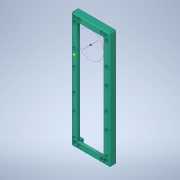
# Autodesk Inventor part: 10_Lid_1x1_v2
Saved by Autodesk Inventor 2022.3 (Build 263350000, 350)
## iProperties
Created: 2019-07-01
Part Number: 10_Lid_1x1_v2
Material: Generic
Document SubType Name: Modeling
Designer: diederichbenedict
Density: 1 g/cm^3
Appearance: IPHT_Türkis
Author: diederichbenedict
Autodesk Inventor part; units mm, degrees
ref_plane "Work Plane1" through (0, 41.8, -12.9) normal (0, 0, 1) x (1, 0, 0)
sketch "Sketch1" plane through (0, 41.8, -12.9) normal (0, 0, 1) x (1, 0, 0)
  line L0 (3.85, 0.3752) -> (3.85, 4) construction
  line L1 (3.85, 4) -> (-2, 4) construction
  arc A0 (-2, 4) -> (-4, 2) centre (-2, 2) ccw construction
  line L2 (-4, 2) -> (-4, -3.85) construction
  line L3 (-4, -3.85) -> (-0.3752, -3.85) construction
  line L4 (-2, 4) -> (43.8, 4)
  line L5 (45.8, 2) -> (45.8, -43.8)
  line L6 (-4, -43.8) -> (-4, 2)
  line L7 (40.3, -37.8) -> (40.3, -4)
  line L8 (37.8, -1.5) -> (4, -1.5)
  line L9 (1.5, -4) -> (1.5, -37.8)
  line L10 (4, -1.5) -> (1.5, -4)
  line L11 (40.3, -4) -> (37.8, -1.5)
  arc A1 (45.8, 2) -> (43.8, 4) centre (43.8, 2) ccw
  arc A2 (-2, 4) -> (-4, 2) centre (-2, 2) ccw
  circle A3 centre (1, -1) radius 1.4
  circle A4 centre (40.8, -1) radius 1.4
  circle A5 centre (40.8, -40.8) radius 1.4 construction
  circle A6 centre (1, -40.8) radius 1.4 construction
  circle A7 centre (20.9, -20.9) radius 19.4 construction
  line L12 (3.85, -3.85) -> (3.85, -37.95)
  line L13 (37.95, -37.95) -> (37.95, -3.85)
  line L14 (37.95, -3.85) -> (3.85, -3.85)
  arc A8 (2.2654, -1.2094) -> (1.2094, -2.2654) centre (0.9, -0.9) ccw projected
  line L15 (2.2654, -1.2094) -> (3.85, 0.3752) projected
  line L16 (-0.3752, -3.85) -> (1.2094, -2.2654) projected
  line L17 (45.8, -47.8) -> (45.8, -93.6)
  line L18 (-4, -93.6) -> (-4, -47.8)
  line L19 (40.3, -87.6) -> (40.3, -53.8)
  line L20 (1.5, -53.8) -> (1.5, -87.6)
  line L21 (40.3, -53.8) -> (37.95, -51.45)
  circle A9 centre (1, -50.8) radius 1.4 construction
  circle A10 centre (40.8, -50.7733) radius 1.4 construction
  circle A11 centre (40.8, -90.6) radius 1.4 construction
  circle A12 centre (1, -90.6) radius 1.4 construction
  circle A13 centre (20.9, -70.7) radius 19.4 construction
  line L22 (3.85, -53.65) -> (3.85, -87.75)
  line L23 (37.95, -87.75) -> (37.95, -53.65)
  line L24 (45.8, -97.6) -> (45.8, -143.4)
  line L25 (43.8, -145.4) -> (-2, -145.4)
  line L26 (-4, -143.4) -> (-4, -97.6)
  line L27 (40.3, -137.4) -> (40.3, -103.6)
  line L28 (1.5, -103.6) -> (1.5, -137.4)
  line L29 (4, -139.9) -> (37.8, -139.9)
  line L30 (37.8, -139.9) -> (40.3, -137.4)
  line L31 (4, -139.9) -> (1.5, -137.4)
  line L32 (40.3, -103.6) -> (37.95, -101.25)
  arc A14 (43.8, -145.4) -> (45.8, -143.4) centre (43.8, -143.4) ccw
  arc A15 (-4, -143.4) -> (-2, -145.4) centre (-2, -143.4) ccw
  circle A16 centre (1, -100.6) radius 1.4 construction
  circle A17 centre (40.8, -100.5154) radius 1.4 construction
  circle A18 centre (40.8, -140.4) radius 1.4
  circle A19 centre (1, -140.4) radius 1.4
  circle A20 centre (20.9, -120.5) radius 19.4 construction
  line L33 (3.85, -103.45) -> (3.85, -137.55)
  line L34 (3.85, -137.55) -> (37.95, -137.55)
  line L35 (37.95, -137.55) -> (37.95, -103.45)
  line L36 (37.95, -37.95) -> (37.95, -40.15)
  line L37 (3.85, -61.4449) -> (3.85, -51.45)
  line L38 (37.95, -37.95) -> (37.95, -40.15)
  line L39 (3.85, -53.65) -> (3.85, -51.45)
  line L40 (3.85, -40.15) -> (3.85, -37.95)
  line L41 (37.95, -40.15) -> (40.3, -37.8)
  line L42 (3.85, -51.45) -> (3.85, -40.15)
  line L43 (3.85, -51.45) -> (3.85, -40.15)
  line L44 (-4, -43.8) -> (-4, -47.8)
  line L45 (45.8, -43.8) -> (45.8, -47.8)
  line L46 (3.85, -40.15) -> (3.85, -37.95)
  line L47 (3.85, -51.45) -> (3.85, -45.8)
  line L48 (37.95, -51.45) -> (37.95, -53.65)
  line L49 (37.95, -40.15) -> (37.95, -51.45)
  line L50 (3.85, -40.15) -> (1.5, -37.8)
  line L51 (3.85, -51.45) -> (1.5, -53.8)
  line L52 (37.95, -40.15) -> (37.95, -51.45)
  line L53 (37.95, -51.45) -> (37.95, -53.65)
  line L54 (37.95, -87.75) -> (37.95, -89.95)
  line L55 (3.85, -87.75) -> (3.85, -89.95)
  line L56 (3.85, -89.95) -> (3.85, -101.25)
  line L57 (3.85, -101.25) -> (1.5, -103.6)
  line L58 (3.85, -101.25) -> (3.85, -103.45)
  line L59 (3.85, -89.95) -> (1.5, -87.6)
  line L60 (37.95, -89.95) -> (37.95, -101.25)
  line L61 (37.95, -89.95) -> (40.3, -87.6)
  line L62 (37.95, -101.25) -> (37.95, -103.45)
  line L63 (-4, -93.6) -> (-4, -97.6)
  line L64 (45.8, -93.6) -> (45.8, -97.6)
  point P0 (45.8, -45.8)
  point P1 (45.8, 4)
  point P2 (-4, -45.8)
  point P3 (40.3, -40.3)
  point P4 (40.3, -1.5)
  point P5 (1.5, -1.5)
  point P6 (1.5, -40.3)
  point P7 (40.8, -1)
  point P8 (45.8, -95.6)
  point P9 (45.8, -45.8)
  point P10 (-4, -95.6)
  point P11 (40.3, -90.1)
  point P12 (40.3, -51.3)
  point P13 (1.5, -51.3)
  point P14 (1.5, -90.1)
  point P15 (40.8, -50.8)
  point P16 (45.8, -145.4)
  point P17 (45.8, -95.6)
  point P18 (-4, -145.4)
  point P19 (40.3, -139.9)
  point P20 (40.3, -101.1)
  point P21 (1.5, -101.1)
  point P22 (1.5, -139.9)
  point P23 (40.8, -100.6)
  point P24 (-0.0387, -1.9387)
  point P25 (1.9387, 0.0387)
  dimension "d55" = 2.8
  dimension "d34" = 49.8
  dimension "d35" = 49.8
  dimension "d36" = 5.5
  dimension "d38" = 2.5
  dimension "d40" = 2.5
  dimension "d41" = 2.5
  dimension "d42" = 2.5
  dimension "d43" = 2.5
  dimension "d44" = 2.5
  dimension "d45" = 2
  dimension "d46" = 5
  dimension "d48" = 5
  dimension "d51" = 5
  dimension "d52" = 0.5
  dimension "d53" = 5
  dimension "d54" = 5
  dimension "d56" = 2.8
  dimension "d57" = 2.8
  dimension "d58" = 2.8
  dimension "d90" = 7.85
  dimension "d112" = 49.8
  dimension "d113" = 49.8
  dimension "d114" = 5.5
  dimension "d116" = 2.5
  dimension "d118" = 2.5
  dimension "d120" = 2.5
  dimension "d121" = 2.5
  dimension "d124" = 5
  dimension "d126" = 5
  dimension "d129" = 0.5
  dimension "d130" = 2.8
  dimension "d131" = 2.8
  dimension "d132" = 2.8
  dimension "d133" = 2.8
  dimension "d134" = 7.85
  dimension "d135" = 49.8
  dimension "d136" = 49.8
  dimension "d137" = 5.5
  dimension "d138" = 2.5
  dimension "d139" = 2.5
  dimension "d140" = 2.5
  dimension "d141" = 2.5
  dimension "d143" = 2.5
  dimension "d144" = 2.5
  dimension "d147" = 5
  dimension "d148" = 5
  dimension "d149" = 5
  dimension "d150" = 5
  dimension "d152" = 0.5
  dimension "d153" = 2.8
  dimension "d154" = 2.8
  dimension "d155" = 2.8
  dimension "d156" = 2.8
  dimension "d157" = 7.85
  constraints: 118 end point, 30 parallel, 30 point on line, 17 centre point, 13 tangent, 9 coincident, 8 point on circle, 4 collinear, 3 perpendicular, 2 vertical, 1 equal radius, 1 horizontal, 1 midpoint, 11 other
  measures "d34" distance of point (45.8, -45.8) point (-4, -45.8)
  measures "d35" distance of point (45.8, 4) point (45.8, -45.8)
  measures "d36" distance between parallel lines of L5 L7
  measures "d38" distance of L7.start point (40.3, -40.3)
  measures "d40" distance of L9.end point (1.5, -40.3)
  measures "d41" distance of L8.end point (1.5, -1.5)
  measures "d42" distance of L9.start point (1.5, -1.5)
  measures "d43" distance of L7.end point (40.3, -1.5)
  measures "d44" distance of L8.start point (40.3, -1.5)
  measures "d45" radius of A1
  measures "d46" distance from line of point (1, -40.8) L6
  measures "d48" distance from line of L5 point (40.8, -40.8)
  measures "d51" distance from line of L4 point (40.8, -1)
  measures "d52" distance from line of point (1, -1) L9
  measures "d53" distance from line of L2 point (1, -1)
  measures "d54" distance from line of L1 point (1, -1)
  measures "d56" diameter of A4
  measures "d57" diameter of A5
  measures "d58" diameter of A6
  measures "d90" distance between parallel lines of L6 L12
  measures "d112" distance of point (45.8, -95.6) point (-4, -95.6)
  measures "d113" distance of point (45.8, -45.8) point (45.8, -95.6)
  measures "d114" distance between parallel lines of L17 L19
  measures "d116" distance of L19.start point (40.3, -90.1)
  measures "d118" distance of L20.end point (1.5, -90.1)
  measures "d120" distance of L20.start point (1.5, -51.3)
  measures "d121" distance of L19.end point (40.3, -51.3)
  measures "d124" distance from line of point (1, -90.6) L18
  measures "d126" distance from line of L17 point (40.8, -90.6)
  measures "d129" distance from line of point (1, -50.8) L20
  measures "d130" diameter of A9
  measures "d131" diameter of A10
  measures "d132" diameter of A11
  measures "d133" diameter of A12
  measures "d134" distance between parallel lines of L18 L22
  measures "d135" distance of point (45.8, -145.4) point (-4, -145.4)
  measures "d136" distance of point (45.8, -95.6) point (45.8, -145.4)
  measures "d137" distance between parallel lines of L24 L27
  measures "d138" distance of L29.end point (40.3, -139.9)
  measures "d139" distance of L27.start point (40.3, -139.9)
  measures "d140" distance of L29.start point (1.5, -139.9)
  measures "d141" distance of L31.end point (1.5, -139.9)
  measures "d143" distance of L28.start point (1.5, -101.1)
  measures "d144" distance of L27.end point (40.3, -101.1)
  measures "d147" distance from line of point (1, -140.4) L26
  measures "d148" distance from line of L25 point (1, -140.4)
  measures "d149" distance from line of L24 point (40.8, -140.4)
  measures "d150" distance from line of L25 point (40.8, -140.4)
  measures "d152" distance from line of point (1, -100.6) L28
  measures "d153" diameter of A16
  measures "d154" diameter of A17
  measures "d155" diameter of A18
  measures "d156" diameter of A19
  measures "d157" distance between parallel lines of L26 L33
extrude "Extrusion1" add sketch "Sketch1" along normal blind 7.7 contours L4 A1 L5 L45 L17 L64 L24 A14 L25 A15 L26 L63 L18 L44 L6 A2 | L41 L36 L13 L14 L12 L40 L50 L9 L10 L8 L11 L7 | L21 L19 L61 L54 L23 L48 | L32 L27 L30 L29 L31 L28 L57 L58 L33 L34 L35 L62 | L37 L22 L55 L59 L20 L51
fillet "Fillet1" radius 2 5 edges at (45.8, -28.9, -5.2) (45.2142, 45.2142, -5.2) (20.9, 45.8, -5.2) (-3.4142, 45.2142, -5.2) (-4, -28.9, -5.2)
sketch "Sketch2" plane through (-2, -4, -12.9) normal (0, -1, 0) x (1, 0, 0)
  line L0 (43.8, -4.8712) -> (42.35, -4)
  line L1 (2, -4.8712) -> (0.55, -4)
  line L2 (-2, 0) -> (-2, 5.7) construction
  line L3 (45.8, 7.7) -> (0, 7.7) construction
  line L4 (47.8, 0) -> (47.8, 5.7) construction
  circle A0 centre (2.9, -62.2) radius 1.45 projected
  line L5 (9.4548, -67.1) -> (36.3452, -67.1) projected
  point P0 (2, 12.9)
  point P1 (2.9, 2.8)
  point P2 (42.9, 2.8)
  dimension "d59" = 4.9
  dimension "d60" = 4.9
  dimension "d61" = 4.9
  dimension "d62" = 4.9
  constraints: 4 end point, 6 other
  measures "d59" distance from line of point (2.9, 2.8) L2
  measures "d60" distance from line of point (2.9, 2.8) L3
  measures "d61" distance from line of point (42.9, 2.8) L4
  measures "d62" distance from line of point (42.9, 2.8) L3
hole "Hole1" [suppressed]
sketch "Sketch3" plane through (0, 41.8, -5.2) normal (0, 0, 1) x (1, 0, 0)
  circle A0 centre (20.9, -20.9) radius 16.9 construction
  point P0 (0, -41.8)
  constraints: 1 centre point
sketch "Sketch4" plane through (0, 41.8, -5.2) normal (0, 0, 1) x (1, 0, 0)
  line L0 (37.95, -37.95) -> (37.95, -3.85) projected
  line L1 (37.95, -3.85) -> (3.85, -3.85) projected
  line L2 (3.85, -3.85) -> (3.85, -37.95) projected
  line L3 (3.85, -37.95) -> (37.95, -37.95) projected
  circle A0 centre (40.9, -0.9) radius 2.75 projected
  circle A1 centre (0.9, -40.9) radius 2.75 projected
  circle A2 centre (0.9, -0.9) radius 2.75 projected
  circle A3 centre (40.9, -40.9) radius 2.75 projected
  line L4 (34.3452, 2) -> (7.4548, 2) projected
  line L5 (43.8, -34.3452) -> (43.8, -7.4548) projected
  line L6 (7.4548, -43.8) -> (34.3452, -43.8) projected
  line L7 (-2, -7.4548) -> (-2, -34.3452) projected
  arc A4 (34.3452, 2) -> (36.4548, 2) centre (35.4, -0.1) ccw projected
  line L8 (43.8, 2) -> (36.4548, 2) projected
  line L9 (43.8, -5.3452) -> (43.8, 2) projected
  arc A5 (43.8, -5.3452) -> (43.8, -7.4548) centre (41.7, -6.4) ccw projected
  arc A6 (43.8, -34.3452) -> (43.8, -36.4548) centre (41.7, -35.4) ccw projected
  line L10 (43.8, -43.8) -> (43.8, -36.4548) projected
  line L11 (36.4548, -43.8) -> (43.8, -43.8) projected
  arc A7 (36.4548, -43.8) -> (34.3452, -43.8) centre (35.4, -41.7) ccw projected
  arc A8 (7.4548, -43.8) -> (5.3452, -43.8) centre (6.4, -41.7) ccw projected
  line L12 (-2, -43.8) -> (5.3452, -43.8) projected
  line L13 (-2, -36.4548) -> (-2, -43.8) projected
  arc A9 (-2, -36.4548) -> (-2, -34.3452) centre (0.1, -35.4) ccw projected
  arc A10 (-2, -7.4548) -> (-2, -5.3452) centre (0.1, -6.4) ccw projected
  line L14 (-2, 2) -> (-2, -5.3452) projected
  line L15 (5.3452, 2) -> (-2, 2) projected
  arc A11 (5.3452, 2) -> (7.4548, 2) centre (6.4, -0.1) ccw projected
  line L16 (37.9698, -87.8712) -> (37.9698, -53.7712)
  line L17 (37.9698, -53.7712) -> (3.8698, -53.7712)
  line L18 (3.8698, -53.7712) -> (3.8698, -87.8712)
  line L19 (3.8698, -87.8712) -> (37.9698, -87.8712)
  circle A12 centre (40.9, -50.8212) radius 2.75
  circle A13 centre (0.9, -90.8212) radius 2.75
  circle A14 centre (0.9, -50.8212) radius 2.75
  circle A15 centre (40.9198, -90.8212) radius 2.75
  line L20 (34.3651, -47.7932) -> (7.4746, -47.7932)
  line L21 (43.8198, -84.1385) -> (43.8198, -57.248)
  line L22 (7.4746, -93.5932) -> (34.3651, -93.5932)
  line L23 (-1.9802, -57.248) -> (-1.9802, -84.1385)
  arc A16 (34.3651, -47.7932) -> (36.4746, -47.7932) centre (35.4198, -49.8932) ccw
  line L24 (43.8198, -47.7932) -> (36.4746, -47.7932)
  line L25 (43.8198, -55.1385) -> (43.8198, -47.7932)
  arc A17 (43.8198, -55.1385) -> (43.8198, -57.248) centre (41.7198, -56.1932) ccw
  arc A18 (43.8198, -84.1385) -> (43.8198, -86.248) centre (41.7198, -85.1932) ccw
  line L26 (43.8198, -93.5932) -> (43.8198, -86.248)
  line L27 (36.4746, -93.5932) -> (43.8198, -93.5932)
  arc A19 (36.4746, -93.5932) -> (34.3651, -93.5932) centre (35.4198, -91.4932) ccw
  arc A20 (7.4746, -93.5932) -> (5.3651, -93.5932) centre (6.4198, -91.4932) ccw
  line L28 (-1.9802, -93.5932) -> (5.3651, -93.5932)
  line L29 (-1.9802, -86.248) -> (-1.9802, -93.5932)
  arc A21 (-1.9802, -86.248) -> (-1.9802, -84.1385) centre (0.1198, -85.1932) ccw
  arc A22 (-1.9802, -57.248) -> (-1.9802, -55.1385) centre (0.1198, -56.1932) ccw
  line L30 (-1.9802, -47.7932) -> (-1.9802, -55.1385)
  line L31 (5.3651, -47.7932) -> (-1.9802, -47.7932)
  arc A23 (5.3651, -47.7932) -> (7.4746, -47.7932) centre (6.4198, -49.8932) ccw
  line L32 (37.9698, -137.5364) -> (37.9698, -103.4364)
  line L33 (3.8698, -103.4364) -> (3.8698, -137.5364)
  line L34 (-1.9802, -107.0412) -> (-1.9802, -133.9317)
  line L35 (37.9698, -103.4364) -> (3.8698, -103.4364)
  line L36 (34.3651, -97.5864) -> (7.4746, -97.5864)
  arc A24 (-1.9802, -107.0412) -> (-1.9802, -104.9317) centre (0.1198, -105.9864) ccw
  arc A25 (5.3651, -97.5864) -> (7.4746, -97.5864) centre (6.4198, -99.6864) ccw
  circle A26 centre (0.9, -100.4864) radius 2.75
  line L37 (5.3651, -97.5864) -> (-1.9802, -97.5864)
  line L38 (-1.9802, -97.5864) -> (-1.9802, -104.9317)
  arc A27 (-1.9802, -136.0412) -> (-1.9802, -133.9317) centre (0.1198, -134.9864) ccw
  line L39 (-1.9802, -136.0412) -> (-1.9802, -143.3864)
  circle A28 centre (0.9, -140.4864) radius 2.75
  line L40 (-1.9802, -143.3864) -> (5.3651, -143.3864)
  arc A29 (7.4746, -143.3864) -> (5.3651, -143.3864) centre (6.4198, -141.2864) ccw
  line L41 (3.8698, -137.5364) -> (37.9698, -137.5364)
  line L42 (7.4746, -143.3864) -> (34.3651, -143.3864)
  circle A30 centre (40.9, -100.4864) radius 2.75
  circle A31 centre (40.9198, -140.4864) radius 2.75
  line L43 (43.8198, -133.9317) -> (43.8198, -107.0412)
  arc A32 (34.3651, -97.5864) -> (36.4746, -97.5864) centre (35.4198, -99.6864) ccw
  line L44 (43.8198, -97.5864) -> (36.4746, -97.5864)
  arc A33 (43.8198, -104.9317) -> (43.8198, -107.0412) centre (41.7198, -105.9864) ccw
  line L45 (43.8198, -104.9317) -> (43.8198, -97.5864)
  arc A34 (36.4746, -143.3864) -> (34.3651, -143.3864) centre (35.4198, -141.2864) ccw
  arc A35 (43.8198, -133.9317) -> (43.8198, -136.0412) centre (41.7198, -134.9864) ccw
  line L46 (36.4746, -143.3864) -> (43.8198, -143.3864)
  line L47 (43.8198, -143.3864) -> (43.8198, -136.0412)
  point P0 (1.6924, -93.5932)
  point P1 (1.6726, -43.8)
  point P2 (1.6924, -47.7932)
  dimension "d159" = 3.9932
  dimension "d160" = 3.9932
  constraints: 64 end point, 32 point on circle, 24 centre point, 4 vertical alignment, 3 midpoint
  measures "d159" vertical distance of point (1.673, -43.8) point (1.692, -47.793)
  measures "d160" distance between parallel lines of L37 L28
hole "Hole2" at (0.9, 40.9, -5.2) at (40.9, 40.9, -5.2) at (40.9198, -98.6864, -5.2) at (0.9, -98.6864, -5.2) direction (0, 0, -1) diameter 3.2 depth 12 tip angle 118 counterbore diameter 6 counterbore depth 3.1
chamfer "Chamfer2" distance 4.6 angle 45 2 edges at (3.85, -28.9, -12.9) (37.95, -28.9, -12.9)
sketch "Sketch6" plane through (-4, -2, -12.9) normal (-1, 0, 0) x (0, 0, 1)
  line L0 (0, -2) -> (5.7, -2) construction
  line L1 (7.7, -99.6) -> (7.7, 45.8) construction
  line L2 (0, 47.8) -> (7.7, 47.8) construction
  circle A0 centre (2.8, 42.9) radius 1.4 construction
  circle A1 centre (2.8, 2.9) radius 1.4 construction
  point P0 (12.9, 2)
  point P1 (7.7, 0)
  point P2 (5.7, 47.8)
  dimension "d63" = 2.8
  dimension "d64" = 2.8
  dimension "d65" = 4.9
  dimension "d66" = 4.9
  dimension "d67" = 4.9
  dimension "d68" = 4.9
  constraints: 2 centre point
  measures "d63" diameter of A0
  measures "d64" diameter of A1
  measures "d65" distance from line of A0.centre L1
  measures "d66" distance from line of A0.centre L2
  measures "d67" distance from line of A1.centre L0
  measures "d68" distance from line of L1 A1.centre
hole "Hole3" [suppressed]
sketch "Sketch7" plane through (45.8, -2, -12.9) normal (1, 0, 0) x (0, 0, -1)
  circle A0 centre (-2.8, 42.9) radius 1.4 projected
  circle A1 centre (-2.8, 2.9) radius 1.4 projected
  point P0 (-12.9, 2)
hole "Hole4" [suppressed]
sketch "Sketch8" plane through (-2, 45.8, -12.9) normal (0, 1, 0) x (1, 0, 0)
  circle A0 centre (2.9, -2.8) radius 1.45 projected
  circle A1 centre (42.9, -2.8) radius 1.45 projected
  point P0 (2, -12.9)
  point P1 (4.35, -2.8)
  point P2 (4.35, -2.8)
  point P3 (44.35, -2.8)
  point P4 (44.35, -2.8)
hole "Hole5" [suppressed]
sketch "Sketch9" plane through (37.95, 3.85, -5.2) normal (-1, 0, 0) x (0, 0, 1)
  line L0 (-7.7, 0) -> (-3.1, 0) projected
  line L1 (-3.1, 34.1) -> (-7.7, 34.1) projected
  line L2 (-3.1, 0) -> (3.4054, 0) construction
  line L3 (-3.1, 34.1) -> (-7.7, 38.7)
  line L4 (-3.1, 34.1) -> (3.4054, 34.1) construction
  line L5 (-7.7, 38.7) -> (-7.7, 34.1)
  line L6 (-7.7, 34.1) -> (-3.1, 34.1)
  line L7 (-3.1, -105.5364) -> (-3.1, -99.5364) projected
  line L8 (-7.7, -99.6) -> (-3.1, -99.6) projected
  line L9 (-3.1, -99.6) -> (-7.7, -99.6)
  line L10 (-7.7, -105.45) -> (-7.7, 39.95) projected
  line L11 (-7.7, -104.2) -> (-3.1, -99.6)
  line L12 (-7.7, 34.1) -> (-7.7, -99.6) projected
  line L13 (-7.7, -104.2) -> (-7.7, -99.6)
  line L14 (-7.7, -99.6) -> (-7.7, -104.2)
  line L15 (-3.1, -99.6) -> (0.0952, -99.6) construction
  point P0 (5.2, -3.85)
  point P1 (-7.7, -5.85)
  point P2 (-7.7, -104.2)
  dimension "d92" = 135
  dimension "d161" = 4.6
  dimension "d162" = 4.6
  dimension "d163" = 135
  constraints: 20 end point, 5 collinear, 3 horizontal, 1 equal length, 1 perpendicular
  measures "d92" angle of L4 L3
  measures "d161" distance of L3.end L1.end
  measures "d162" distance of L8.start L11.start
  measures "d163" angle of L15 L11
extrude "Extrusion3" cut sketch "Sketch9" along normal up to surface (34.1 mm away)
sketch "Sketch13" plane through (0, 41.8, -5.2) normal (0, 0, 1) x (1, 0, 0)
  circle A0 centre (32.9, -28) radius 0.5 construction
  circle A1 centre (32.9, -26) radius 0.5 construction
  circle A2 centre (32.9, -24) radius 0.5 construction
  circle A3 centre (32.9, -22) radius 0.5 construction
  circle A4 centre (32.9, -20) radius 0.5 construction
  circle A5 centre (32.9, -18) radius 0.5 construction
  circle A6 centre (32.9, -16) radius 0.5 construction
  circle A7 centre (32.9, -14) radius 0.5 construction
  circle A8 centre (32.9, -12) radius 0.5 construction
  circle A9 centre (32.9, -10) radius 0.5 construction
  circle A10 centre (34.9, -28) radius 0.5 construction
  circle A11 centre (34.9, -26) radius 0.5 construction
  circle A12 centre (34.9, -24) radius 0.5 construction
  circle A13 centre (34.9, -22) radius 0.5 construction
  circle A14 centre (34.9, -20) radius 0.5 construction
  circle A15 centre (34.9, -18) radius 0.5 construction
  circle A16 centre (34.9, -16) radius 0.5 construction
  circle A17 centre (34.9, -14) radius 0.5 construction
  circle A18 centre (34.9, -12) radius 0.5 construction
  circle A19 centre (34.9, -10) radius 0.5 construction
  circle A20 centre (9.1, -28) radius 0.5 construction
  circle A21 centre (9.1, -26) radius 0.5 construction
  circle A22 centre (9.1, -24) radius 0.5 construction
  circle A23 centre (9.1, -22) radius 0.5 construction
  circle A24 centre (9.1, -20) radius 0.5 construction
  circle A25 centre (9.1, -18) radius 0.5 construction
  circle A26 centre (9.1, -16) radius 0.5 construction
  circle A27 centre (9.1, -14) radius 0.5 construction
  circle A28 centre (9.1, -12) radius 0.5 construction
  circle A29 centre (9.1, -10) radius 0.5 construction
  circle A30 centre (7.1, -28) radius 0.5 construction
  circle A31 centre (7.1, -26) radius 0.5 construction
  circle A32 centre (7.1, -24) radius 0.5 construction
  circle A33 centre (7.1, -22) radius 0.5 construction
  circle A34 centre (7.1, -20) radius 0.5 construction
  circle A35 centre (7.1, -18) radius 0.5 construction
  circle A36 centre (7.1, -16) radius 0.5 construction
  circle A37 centre (7.1, -14) radius 0.5 construction
  circle A38 centre (7.1, -12) radius 0.5 construction
  circle A39 centre (7.1, -10) radius 0.5 construction
  line L0 (25.3, -35.4) -> (25.3, -39) construction
  line L1 (25.3, -39) -> (25.6, -39) construction
  line L2 (25.6, -39) -> (25.6, -41) construction
  line L3 (25.6, -41) -> (36.6, -41) construction
  line L4 (36.6, -41) -> (36.6, -4) construction
  line L5 (36.6, -4) -> (34.6, -2) construction
  line L6 (34.6, -2) -> (7.4, -2) construction
  line L7 (7.4, -2) -> (5.4, -4) construction
  line L8 (5.4, -4) -> (5.4, -34.7) construction
  line L9 (5.4, -34.7) -> (8, -34.7) construction
  line L10 (8, -34.7) -> (8, -35.4) construction
  line L11 (8, -35.4) -> (10.0553, -35.4) construction
  line L12 (10.0553, -35.4) -> (10.0553, -40.4269) construction
  line L13 (10.0553, -40.4269) -> (8, -40.4269) construction
  line L14 (8, -40.4269) -> (8, -41) construction
  line L15 (8, -41) -> (16.3, -41) construction
  line L16 (16.3, -41) -> (16.3, -39) construction
  line L17 (16.3, -39) -> (17.1, -39) construction
  line L18 (17.1, -39) -> (17.1, -35.4) construction
  line L19 (17.1, -35.4) -> (25.3, -35.4) construction
  line L20 (13, -9.2) -> (28.5, -9.2) construction
  line L21 (28.5, -9.2) -> (28.5, -26.7) construction
  line L22 (28.5, -26.7) -> (13, -26.7) construction
  line L23 (13, -26.7) -> (13, -9.2) construction
  line L24 (7.1929, -1.5) -> (34.8071, -1.5)
  line L25 (34.8071, -1.5) -> (37.1, -3.7929)
  line L26 (37.1, -3.7929) -> (37.1, -41.5)
  line L27 (37.1, -41.5) -> (25.1, -41.5)
  line L28 (25.1, -41.5) -> (25.1, -39.5)
  line L29 (25.1, -39.5) -> (24.8, -39.5)
  line L30 (24.8, -39.5) -> (24.8, -35.9)
  line L31 (24.8, -35.9) -> (17.6, -35.9)
  line L32 (17.6, -35.9) -> (17.6, -39.5)
  line L33 (17.6, -39.5) -> (16.8, -39.5)
  line L34 (16.8, -39.5) -> (16.8, -41.5)
  line L35 (16.8, -41.5) -> (7.5, -41.5)
  line L36 (7.5, -41.5) -> (7.5, -39.9269)
  line L37 (7.5, -39.9269) -> (9.5553, -39.9269)
  line L38 (9.5553, -39.9269) -> (9.5553, -35.9)
  line L39 (9.5553, -35.9) -> (7.5, -35.9)
  line L40 (7.5, -35.9) -> (7.5, -35.2)
  line L41 (7.5, -35.2) -> (4.9, -35.2)
  line L42 (4.9, -35.2) -> (4.9, -3.7929)
  line L43 (4.9, -3.7929) -> (7.1929, -1.5)
  line L44 (4.9, -8.3094) -> (-7.5, -8.3094)
  line L45 (-7.5, -8.3094) -> (-7.5, -29.6022)
  line L46 (-7.5, -29.6022) -> (4.9, -29.6022)
  line L47 (4.9, -29.6022) -> (4.9, -8.3094)
  line L48 (37.1, -8.3094) -> (50.916, -8.3094)
  line L49 (50.916, -8.3094) -> (50.916, -29.6022)
  line L50 (50.916, -29.6022) -> (37.1, -29.6022)
  line L51 (37.1, -29.6022) -> (37.1, -8.3094)
  line L52 (9.5553, -39.9269) -> (4.9, -39.9269)
  line L53 (4.9, -39.9269) -> (4.9, -35.2)
  line L54 (4.9, -35.2) -> (9.5553, -35.2)
  line L55 (9.5553, -35.2) -> (9.5553, -39.9269)
  line L56 (15, -35.2) -> (26.8, -35.2)
  line L57 (26.8, -35.2) -> (26.8, -46.7944)
  line L58 (26.8, -46.7944) -> (15, -46.7944)
  line L59 (15, -46.7944) -> (15, -35.2)
  line L60 (-4, 2) -> (-4, -143.4) projected
  line L61 (45.8, -143.4) -> (45.8, 2) projected
  point P0 (0, -41.8)
  point P1 (-4, -43.8)
  point P2 (45.8, -43.8)
  dimension "d100" = 0.5
  dimension "d101" = 19
  dimension "d102" = 19
  constraints: 72 end point, 8 parallel, 4 horizontal, 4 perpendicular, 3 point on line, 1 collinear, 19 other
  measures "d100" distance between parallel lines of L6 L24
  measures "d101" distance between parallel lines of L60 L59
  measures "d102" distance between parallel lines of L61 L57
ref_plane "Work Plane2" through (5.4, 0.8, 6) normal (0, 0, 1) x (1, 0, 0)
ref_plane "Work Plane3" through (5.4, 0.8, 5) normal (0, 0, -1) x (0, 1, 0)
sketch "Sketch14" plane through (0, 41.8, -5.2) normal (0, 0, 1) x (1, 0, 0)
  arc A0 (40.1319, 2) -> (43.8, -1.6681) centre (40.9, -0.9) ccw construction
  arc A1 (-2, -1.6681) -> (1.6681, 2) centre (0.9, -0.9) ccw construction
  line L0 (43.8, -143.4) -> (41.6347, -143.4) projected
  line L1 (43.8, -1.6681) -> (43.8, -139.6471) projected
  line L2 (1.6681, 2) -> (40.1319, 2) projected
  line L3 (-2, -139.7183) -> (-2, -1.6681) projected
  line L4 (3.85, -137.55) -> (3.85, -3.85) projected
  line L5 (3.85, -3.85) -> (37.95, -3.85) projected
  line L6 (37.95, -3.85) -> (37.95, -137.55) projected
  line L7 (37.95, -137.55) -> (3.85, -137.55) projected
  arc A2 (1.6149, -143.4) -> (-2, -139.7183) centre (0.9, -140.4864) ccw projected
  line L8 (40.2049, -143.4) -> (1.6149, -143.4) projected
  arc A3 (43.8, -139.6471) -> (40.2049, -143.4) centre (40.9198, -140.4864) ccw projected
  arc A4 (-2, -141.2545) -> (0.1851, -143.4) centre (0.9, -140.4864) ccw projected
  line L9 (-2, -143.4) -> (-2, -141.2545) projected
  line L10 (0.1851, -143.4) -> (-2, -143.4) projected
  arc A5 (43.8, -0.1319) -> (41.6681, 2) centre (40.9, -0.9) ccw projected
  line L11 (43.8, 2) -> (43.8, -0.1319) projected
  line L12 (41.6681, 2) -> (43.8, 2) projected
  arc A6 (0.1319, 2) -> (-2, -0.1319) centre (0.9, -0.9) ccw projected
  line L13 (-2, 2) -> (0.1319, 2) projected
  line L14 (-2, -0.1319) -> (-2, 2) projected
  arc A7 (41.6347, -143.4) -> (43.8, -141.3258) centre (40.9198, -140.4864) ccw projected
  line L15 (43.8, -141.3258) -> (43.8, -143.4) projected
  point P0 (0, -41.8)
  point P1 (6.4, -0.1)
  point P2 (0.1, -6.4)
  point P3 (0.1, -35.4)
  point P4 (6.4, -41.7)
  point P5 (35.4, -41.7)
  point P6 (41.7, -35.4)
  point P7 (41.7, -6.4)
  point P8 (35.4, -0.1)
  point P9 (41.7, -56.3212)
  point P10 (41.7, -85.3212)
  point P11 (41.7, -105.9864)
  point P12 (41.7, -134.9864)
  point P13 (35.4198, -141.3)
  point P14 (6.3395, -141.3)
  point P15 (0.1, -134.9864)
  point P16 (0.1, -105.9864)
  point P17 (0.1, -85.3212)
  point P18 (0.1, -56.3212)
  dimension "d164" = 5.5
  dimension "d165" = 5.5
  dimension "d166" = 2.1
  dimension "d167" = 2.1
  dimension "d172" = 5.5
  dimension "d176" = 5.5
  dimension "d177" = 5.5
  dimension "d178" = 5.5
  dimension "d179" = 2.1
  dimension "d180" = 2.1
  constraints: 7 vertical alignment
  measures "d164" vertical distance of A0.centre point (41.7, -6.4)
  measures "d165" horizontal distance of A0.centre point (35.4, -0.1)
  measures "d166" distance from line of L2 point (35.4, -0.1)
  measures "d167" distance from line of L1 point (41.7, -35.4)
  measures "d172" vertical distance of point (41.7, -134.986) A7.centre
  measures "d176" vertical distance of point (0.1, -134.986) A2.centre
  measures "d177" distance of point (6.339, -141.3) A2.centre
  measures "d178" horizontal distance of A7.centre point (35.42, -141.3)
  measures "d179" distance from line of point (6.339, -141.3) L8
  measures "d180" distance from line of L8 point (35.42, -141.3)
hole "Hole6" at (6.4, 41.7, -5.2) at (0.1, 35.4, -5.2) at (0.1, 6.4, -5.2) at (6.4, 0.1, -5.2) at (35.4, 0.1, -5.2) at (41.7, 6.4, -5.2) at (41.7, 35.4, -5.2) at (35.4, 41.7, -5.2) at (0.1, -14.5212, -5.2) at (41.7, -14.5212, -5.2) at (41.7, -43.5212, -5.2) at (41.7, -64.1864, -5.2) at (0.1, -43.5212, -5.2) at (0.1, -64.1864, -5.2) at (0.1, -93.1864, -5.2) at (6.3395, -99.5, -5.2) at (35.4198, -99.5, -5.2) at (41.7, -93.1864, -5.2) direction (0, 0, -1) diameter 4.7 end through all
equation "\"d38\" = d37"
equation "\"d40\" = d39"
equation "\"d41\" = d37"
equation "\"d42\" = d41"
equation "\"d43\" = d37"
equation "\"d44\" = d43"
equation "\"d39\" = d37"
equation "\"d37\" = 2.5"
body "Solid1"
